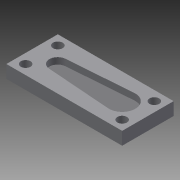
# Autodesk Inventor part: ServoHornHolder
Saved by Autodesk Inventor 2015 (Build 190159000, 159)
## iProperties
Created: 2014-09-29
Part Number: ServoHornHolder
Material: Generic
Document SubType Name: Modeling
Designer: Jaden
Density: 1 g/cm^3
Appearance: Default
Author: Jaden
Autodesk Inventor part; units mm, degrees
ref_plane "YZ Plane" through (0, 0, 0) normal (1, 0, 0) x (0, 1, 0)
ref_plane "XZ Plane" through (0, 0, 0) normal (0, 1, 0) x (-1, 0, 0)
ref_plane "XY Plane" through (0, 0, 0) normal (0, 0, 1) x (1, 0, 0)
sketch "Sketch1" plane through (0, 0, 0) normal (0, 0, 1) x (1, 0, 0)
  line L0 (-12.7, 28.575) -> (12.7, 28.575)
  line L1 (12.7, 28.575) -> (12.7, -28.575)
  line L2 (12.7, -28.575) -> (-12.7, -28.575)
  line L3 (-12.7, -28.575) -> (-12.7, 28.575)
  point P0 (0, 0)
  point P1 (12.7, 0)
  point P2 (0, 28.575)
  dimension "d0" = 25.4
  dimension "d1" = 57.15
  constraints: 8 end point, 2 midpoint, 2 parallel, 1 horizontal, 1 horizontal alignment, 1 perpendicular, 1 vertical alignment
  measures "d0" distance of L0.start L0.end
  measures "d1" distance of L0.end L1.end
extrude "Extrusion1" add sketch "Sketch1" along normal blind 6.35
sketch "Sketch2" plane through (0, 0, 6.35) normal (0, 0, 1) x (1, 0, 0)
  arc A0 (-6.4964, -15.3835) -> (6.4964, -15.3835) centre (0, -15.875) ccw
  arc A1 (4.1031, 16.2496) -> (-4.1031, 16.2496) centre (0, 15.9392) ccw
  line L0 (4.1031, 16.2496) -> (6.4964, -15.3835)
  line L1 (-4.1031, 16.2496) -> (-6.4964, -15.3835)
  line L2 (-12.7, -28.575) -> (12.7, -28.575) projected
  line L3 (12.7, -28.575) -> (12.7, 28.575) projected
  dimension "d12" = 4.1148
  dimension "d13" = 6.515
  dimension "d18" = 4.327
  dimension "d23" = 12.7
  dimension "d54" = 31.8142
  dimension "d55" = 6.185
  constraints: 4 end point, 4 point on circle, 4 tangent, 2 centre point
  measures "d12" radius of A1
  measures "d13" radius of A0
  measures "d18" angle of L0 L3
  measures "d23" distance from line of L3 A0.centre
  measures "d54" distance of A0.centre A1.centre
  measures "d55" distance edge to line of A0 L2
extrude "Extrusion2" cut sketch "Sketch2" against normal blind 3.175
sketch "Sketch4" plane through (0, 0, 6.35) normal (0, 0, 1) x (1, 0, 0)
  line L0 (7.9375, 23.8125) -> (-7.9375, 23.8125)
  line L1 (-7.9375, 23.8125) -> (-7.9375, -23.8125)
  line L2 (-7.9375, -23.8125) -> (7.9375, -23.8125)
  line L3 (7.9375, -23.8125) -> (7.9375, 23.8125)
  line L4 (12.7, 28.575) -> (12.7, -28.575) projected
  line L5 (-12.7, -28.575) -> (12.7, -28.575) projected
  point P0 (0, 0)
  dimension "d42" = 4.7625
  dimension "d43" = 4.7625
  dimension "d44" = 47.625
  dimension "d45" = 15.875
  constraints: 8 end point, 2 parallel, 1 horizontal, 1 perpendicular
  measures "d42" distance between parallel lines of L4 L3
  measures "d43" distance between parallel lines of L5 L2
  measures "d44" distance of L0.end L1.end
  measures "d45" distance of L0.start L0.end
hole "Hole1" at (7.9375, 23.8125, 6.35) at (-7.9375, 23.8125, 6.35) at (-7.9375, -23.8125, 6.35) at (7.9375, -23.8125, 6.35) direction (0, 0, -1) diameter 4.7625 end through all
equation "\"d0\" = plate_width"
equation "\"d1\" = plate_height"
equation "\"d23\" = 0.5 * plate_width"
equation "\"d54\" = slot_centers"
equation "\"d42\" = hole_dist"
equation "\"d43\" = hole_dist"
equation "\"d44\" = plate_height - 2 * hole_dist"
equation "\"d45\" = plate_width - 2 * hole_dist"
equation "\"d46\" = hole_dia"
equation "\"plate_width\" = 25.4"
equation "\"plate_height\" = 57.15"
equation "\"slot_centers\" = 31.81417"
equation "\"hole_dia\" = 4.7625"
equation "\"hole_dist\" = 4.7625"
body "Solid1"
